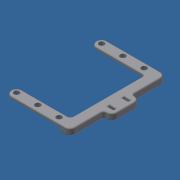
# Autodesk Inventor part: MotorServo2
Saved by Autodesk Inventor 2015 SP1 (Build 190203100, 203)
## iProperties
Created: 2015-11-11
Part Number: MotorServo2
Material: Generic
Document SubType Name: Modeling
Designer: Dale
Density: 1 g/cm^3
Appearance: Default
Author: Dale
Autodesk Inventor part; units mm, degrees
ref_plane "YZ Plane" through (0, 0, 0) normal (1, 0, 0) x (0, 1, 0)
ref_plane "XZ Plane" through (0, 0, 0) normal (0, 1, 0) x (-1, 0, 0)
ref_plane "XY Plane" through (0, 0, 0) normal (0, 0, 1) x (1, 0, 0)
sketch "Sketch1" plane through (0, 0, 0) normal (0, 0, 1) x (1, 0, 0)
  line L0 (-20.5, -32) -> (-20.5, -32)
  line L1 (-16.5, -28) -> (18, -28)
  line L2 (20, -26) -> (20, 26)
  line L3 (18, 28) -> (-16.5, 28)
  line L4 (-20.5, 32) -> (-20.5, 32)
  line L5 (-16.5, 36) -> (24, 36)
  line L6 (28, 32) -> (28, 12.5)
  line L7 (30, 10.5) -> (30, 10.5)
  line L8 (34, 6.5) -> (34, -6.5)
  line L9 (30, -10.5) -> (30, -10.5)
  line L10 (28, -12.5) -> (28, -32)
  line L11 (24, -36) -> (-16.5, -36)
  arc A0 (-20.5, -32) -> (-16.5, -36) centre (-16.5, -32) ccw
  arc A1 (24, -36) -> (28, -32) centre (24, -32) ccw
  arc A2 (-16.5, 36) -> (-20.5, 32) centre (-16.5, 32) ccw
  arc A3 (28, 32) -> (24, 36) centre (24, 32) ccw
  arc A4 (20, 26) -> (18, 28) centre (18, 26) ccw
  arc A5 (28, 12.5) -> (30, 10.5) centre (30, 12.5) ccw
  arc A6 (30, -10.5) -> (28, -12.5) centre (30, -12.5) ccw
  arc A7 (18, -28) -> (20, -26) centre (18, -26) ccw
  arc A8 (34, 6.5) -> (30, 10.5) centre (30, 6.5) ccw
  arc A9 (30, -10.5) -> (34, -6.5) centre (30, -6.5) ccw
  arc A10 (-16.5, -28) -> (-20.5, -32) centre (-16.5, -32) ccw
  arc A11 (-20.5, 32) -> (-16.5, 28) centre (-16.5, 32) ccw
  point P0 (0, 0)
  point P1 (-20.5, 28)
  point P2 (-20.5, 36)
  point P3 (28, 10.5)
  point P4 (34, 10.5)
  point P5 (28, -10.5)
  point P6 (28, -36)
  dimension "d0" = 72
  dimension "d1" = 36
  dimension "d2" = 48.5
  dimension "d3" = 40.5
  dimension "d5" = 20
  dimension "d6" = 8
  dimension "d7" = 8
  dimension "d8" = 6
  dimension "d9" = 25.5
  dimension "d11" = 4
  dimension "d12" = 2
  dimension "d13" = 4
  dimension "d14" = 4
  dimension "d53" = 21
  constraints: 24 end point, 24 point on circle, 24 tangent, 16 point on line, 12 centre point, 8 equal radius, 6 horizontal, 4 vertical
  measures "d0" distance between parallel lines of L11 L5
  measures "d1" distance from line of point (0, 0) L5
  measures "d2" distance between parallel lines of L6 L4
  measures "d3" distance between parallel lines of L2 L4
  measures "d5" distance from line of point (0, 0) L2
  measures "d6" distance between parallel lines of L11 L1
  measures "d7" distance between parallel lines of L3 L5
  measures "d8" distance of point (28, 10.5) point (34, 10.5)
  measures "d9" distance between parallel lines of L11 L9
  measures "d11" radius of A0
  measures "d12" radius of A4
  measures "d13" radius of A8
  measures "d14" radius of A10
  measures "d53" distance of L7.start L9.end
extrude "Base" add sketch "Sketch1" along normal blind 5.2
sketch "Sketch2" plane through (0, 0, 5.2) normal (0, 0, 1) x (1, 0, 0)
  circle A0 centre (-16.5, -32) radius 2.05
  line L0 (-16.5, -36) -> (24, -36) projected
  line L1 (34, -10.5) -> (34, 6.5) construction
  circle A1 centre (-0.5, -32) radius 2.05
  circle A2 centre (15.5, -32) radius 2.05
  circle A3 centre (-16.5, 32) radius 2.05
  circle A4 centre (-0.5, 32) radius 2.05
  circle A5 centre (15.5, 32) radius 2.05
  line L2 (-20.5, -28) -> (-20.5, -36) construction
  arc A6 (-16.5, -28) -> (-16.5, -36) centre (-16.5, -32) ccw construction
  point P0 (0, 0)
  point P1 (30, -10.5)
  dimension "d17" = 4.1
  dimension "d18" = 4
  dimension "d22" = 16
  dimension "d25" = 64
  dimension "d58" = 4
  constraints: 6 centre point, 4 end point, 3 horizontal alignment, 3 vertical, 1 horizontal, 1 tangent, 10 other
  measures "d17" diameter of A0
  measures "d18" distance from line of A0.centre L0
  measures "d22" distance of A0.centre A1.centre
  measures "d25" distance of A0.centre A3.centre
  measures "d58" distance from line of L2 A0.centre
extrude "Mounting Holes" cut sketch "Sketch2" against normal through all
sketch "Sketch3" plane through (0, 0, 5.2) normal (0, 0, 1) x (1, 0, 0)
  line L0 (26.5, -4.5) -> (31, -4.5)
  line L1 (31, -4.5) -> (31, -6.5)
  line L2 (31, -6.5) -> (26.5, -6.5)
  line L3 (26.5, -6.5) -> (26.5, -4.5)
  line L4 (-16.5, -36) -> (24, -36) projected
  line L5 (20, 26) -> (20, -26) projected
  line L6 (26.5, 6.5) -> (31, 6.5)
  line L7 (31, 6.5) -> (31, 4.5)
  line L8 (31, 4.5) -> (26.5, 4.5)
  line L9 (26.5, 4.5) -> (26.5, 6.5)
  arc A0 (30, -10.5) -> (28, -12.5) centre (30, -12.5) ccw projected
  line L10 (24, 36) -> (-16.5, 36) projected
  point P0 (0, 0)
  dimension "d32" = 2
  dimension "d33" = 4.5
  dimension "d34" = 6.5
  dimension "d37" = 11
  dimension "d55" = 4
  constraints: 16 end point, 2 parallel, 1 horizontal, 1 perpendicular, 1 vertical, 8 other
  measures "d32" distance between parallel lines of L2 L0
  measures "d33" distance of L1.end L2.end
  measures "d34" distance between parallel lines of L3 L5
  measures "d37" distance of L0.start L6.start
  measures "d55" distance from line of L2 A0.start
extrude "Zip Tie Slot" cut sketch "Sketch3" against normal through all
sketch "Sketch4" plane through (0, 0, 0) normal (0, 0, -1) x (-1, 0, 0)
  line L0 (16.5, 36) -> (-24, 36) projected
  line L1 (-20, 36) -> (20.5, 36)
  line L2 (20.5, 36) -> (20.5, -36)
  line L3 (20.5, -36) -> (-20, -36)
  line L4 (-20, -36) -> (-20, 36)
  line L5 (-24, -36) -> (16.5, -36) projected
  line L6 (-20, -26) -> (-20, 26) projected
  arc A0 (16.5, 36) -> (16.5, 36) centre (16.5, 32) ccw projected
  point P0 (0, 0)
  point P1 (20, 40)
  constraints: 8 end point, 2 collinear, 2 parallel, 1 horizontal, 1 perpendicular, 1 point on line, 1 vertical, 1 other
extrude "Mount Cutout" cut sketch "Sketch4" against normal blind 3
sketch "Sketch5" plane through (0, 0, 0) normal (0, 0, -1) x (-1, 0, 0)
  line L0 (-31, 4.5) -> (-26.5, 4.5)
  line L1 (-26.5, 4.5) -> (-26.5, -4.5)
  line L2 (-26.5, -4.5) -> (-31, -4.5)
  line L3 (-31, -4.5) -> (-31, 4.5)
  line L4 (-26.5, 4.5) -> (-31, 4.5) projected
  line L5 (-31, 4.5) -> (-31, 6.5) projected
  point P0 (0, 0)
  constraints: 8 end point, 2 collinear, 2 parallel, 1 horizontal, 1 perpendicular
extrude "Zip Tie Cutout" cut sketch "Sketch5" against normal blind 2
fillet "Rounded Zip Tie Strap" radius 2 2 edges at (28.75, -4.5, 2) (28.75, 4.5, 2)
fillet "Rounded Cutout" radius 0.8 4 edges at (28.75, 6.5, 0) (31, 0, 0) (28.75, -6.5, 0) (26.5, 0, 0)
fillet "Rounded Top" radius 1 18 edges at (20, 0, 5.2) (19.4142, -27.4142, 5.2) (0.75, -28, 5.2) (-20.5, -32, 5.2) (3.75, -36, 5.2) (26.8284, -34.8284, 5.2) (28, -22.25, 5.2) (28.5858, -11.0858, 5.2) (32.8284, -9.3284, 5.2) (34, 0, 5.2) (32.8284, 9.3284, 5.2) (28.5858, 11.0858, 5.2) (28, 22.25, 5.2) (26.8284, 34.8284, 5.2) (3.75, 36, 5.2) (-20.5, 32, 5.2) (0.75, 28, 5.2) (19.4142, 27.4142, 5.2)
fillet "Rounded Bottom" radius 1 11 edges at (28, 22.25, 0) (26.8284, 34.8284, 0) (22, 36, 0) (28.5858, 11.0858, 0) (32.8284, 9.3284, 0) (34, 0, 0) (32.8284, -9.3284, 0) (28.5858, -11.0858, 0) (28, -22.25, 0) (26.8284, -34.8284, 0) (22, -36, 0)
fillet "Rounded Slots" radius 0.8 8 edges at (28.75, 6.5, 5.2) (31, 5.5, 5.2) (28.75, 4.5, 5.2) (26.5, 5.5, 5.2) (28.75, -4.5, 5.2) (28.75, -6.5, 5.2) (31, -5.5, 5.2) (26.5, -5.5, 5.2)
body "Solid1"
